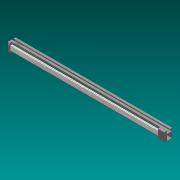
# Autodesk Inventor part: 连接桥
Saved by Autodesk Inventor 2021 (Build 250183000, 183)
## iProperties
Created: 2025-04-17
Part Number: 连接桥
Material: 常规
Document SubType Name: Modeling
Designer: 86155
Density: 1 g/cm^3
Appearance: 默认
Author: 86155
Autodesk Inventor part; units mm, degrees
ref_plane "YZ Plane" through (0, 0, 0) normal (1, 0, 0) x (0, 1, 0)
ref_plane "XZ Plane" through (0, 0, 0) normal (0, 1, 0) x (-1, 0, 0)
ref_plane "XY Plane" through (0, 0, 0) normal (0, 0, 1) x (1, 0, 0)
sketch "草图1" plane through (0, 0, 0) normal (1, 0, 0) x (0, 1, 0)
  line L0 (21, 12.5) -> (-21, 12.5)
  line L1 (-21, 12.5) -> (-21, -12.5)
  line L2 (-21, -12.5) -> (21, -12.5)
  line L3 (21, 12.5) -> (-21, -12.5) construction
  line L4 (-21, 12.5) -> (21, -12.5) construction
  line L5 (19, 10.5) -> (-19, 10.5)
  line L6 (-19, 10.5) -> (-19, -10.5)
  line L7 (-19, -10.5) -> (19, -10.5)
  line L8 (21, 4.5) -> (19, 4.5)
  line L9 (21, -4.5) -> (19, -4.5)
  line L10 (21, -12.5) -> (21, -4.5)
  line L11 (21, 4.5) -> (21, 12.5)
  line L12 (19, -10.5) -> (19, -4.5)
  line L13 (19, 4.5) -> (19, 10.5)
  line L14 (0, 10.5) -> (-2, 10.5)
  line L15 (-2, -10.5) -> (0, -10.5)
  line L16 (8, -12.5) -> (6, -12.5)
  line L17 (6, -12.5) -> (6, 12.5)
  line L18 (6, 12.5) -> (8, 12.5)
  line L19 (8, 12.5) -> (8, -12.5)
  point P0 (0, 0)
  point P1 (6, -10.5)
  point P2 (6, 10.5)
  point P3 (8, -10.5)
  point P4 (8, 10.5)
  dimension "d0" = 42
  dimension "d1" = 25
  dimension "d3" = 8
  dimension "d4" = 8
  dimension "d9" = 2
  dimension "d10" = 25
  constraints: 40 end point, 9 parallel, 7 perpendicular, 3 horizontal, 3 midpoint, 3 point on line, 2 other
  measures "d0" distance of L2.end L1.end
  measures "d1" distance of L1.end L0.end
  measures "d3" distance between parallel lines of L2 L9
  measures "d4" distance between parallel lines of L0 L8
  measures "d9" distance of L17.end L18.end
  measures "d10" distance between parallel lines of L6 L17
extrude "拉伸2" add sketch "草图1" along normal blind 680 contours L11 L8 L13 L5 L19 L0 | L19 L5 L17 L0 | L17 L5 L6 L7 L2 L1 L0 | L19 L7 L17 L5 | L19 L2 L17 L7 | L7 L12 L9 L10 L2 L19
sketch "草图2" plane through (0, -19, -10.5) normal (0, 0, 1) x (1, 0, 0)
  circle A0 centre (617.3314, 19) radius 3.3235 projected
  circle A1 centre (647.3314, 19) radius 3.3235 projected
  point P0 (0, 19)
extrude "拉伸3" cut sketch "草图2" against normal blind 2
sketch "草图3" plane through (0, 0, 0) normal (-1, 0, 0) x (0, 0, 1)
  line L0 (-12.5, 21) -> (-4.5, 21) projected
  line L1 (-12.5, -21) -> (-12.5, 21) projected
  line L2 (12.5, -21) -> (-12.5, -21) projected
  line L3 (12.5, 21) -> (12.5, -21) projected
  line L4 (4.5, 21) -> (12.5, 21) projected
  line L5 (4.5, 19) -> (4.5, 21) projected
  line L6 (10.5, 19) -> (4.5, 19) projected
  line L7 (10.5, 8) -> (10.5, 19) projected
  line L8 (-10.5, 8) -> (10.5, 8) projected
  line L9 (-10.5, 19) -> (-10.5, 8) projected
  line L10 (-4.5, 19) -> (-10.5, 19) projected
  line L11 (-4.5, 21) -> (-4.5, 19) projected
  line L12 (-10.5, 6) -> (-10.5, -19) projected
  line L13 (10.5, 6) -> (-10.5, 6) projected
  line L14 (10.5, -19) -> (10.5, 6) projected
  line L15 (-10.5, -19) -> (10.5, -19) projected
  line L16 (-10.5, 8) -> (-10.5, 6)
  line L17 (-10.5, 8) -> (10.5, 8) projected
  line L18 (10.5, -19) -> (10.5, 6) projected
  line L19 (10.5, 8) -> (10.5, 6)
  point P0 (0, 0)
  constraints: 4 end point, 1 collinear
extrude "拉伸4" add sketch "草图3" along normal blind 40 contours L0 L11 L10 L9 L16 L12 L15 L14 L19 L7 L6 L5 L4 L3 L2 L1
sketch "草图4" plane through (680, -21, 12.5) normal (0, 0, 1) x (1, 0, 0)
  circle A0 centre (-698, 21) radius 4.25
  line L0 (-720, 0) -> (-720, 42) projected
  point P0 (-680, 21)
  dimension "d17" = 8.5
  dimension "d18" = 22
  constraints: 1 centre point
  measures "d17" diameter of A0
  measures "d18" distance from line of L0 A0.centre
extrude "拉伸5" cut sketch "草图4" against normal blind 40
sketch "草图5" plane through (-40, 0, 0) normal (-1, 0, 0) x (0, 0, 1)
  line L0 (4.5, 21) -> (12.5, 21) projected
  line L1 (12.5, 21) -> (22.5, 21)
  line L2 (22.5, 21) -> (22.5, -21)
  line L3 (22.5, -21) -> (12.5, -21)
  line L4 (12.5, -21) -> (12.5, 21)
  point P0 (0, 0)
  dimension "d21" = 10
  dimension "d22" = 42
  constraints: 8 end point, 2 parallel, 1 horizontal, 1 perpendicular
  measures "d21" distance of L2.end L3.end
  measures "d22" distance of L1.end L2.end
extrude "拉伸6" add sketch "草图5" against normal blind 10
chamfer "倒角1" distance 2 angle 45 2 edges at (-35, 21, 22.5) (-35, -21, 22.5)
sketch "草图6" plane through (-30, 0, 0) normal (1, 0, 0) x (0, 0, -1)
  line L0 (-12.5, 21) -> (-12.5, -21) projected
  line L1 (-20.5, -10) -> (-20.5, 10)
  line L2 (-12.5, 10) -> (-12.5, -10)
  line L3 (-12.5, 21) -> (-20.5, 21) projected
  line L4 (-15.5, -10) -> (-15.5435, -10)
  line L5 (-15.5, -10) -> (-17.5, -10)
  line L6 (-17.5, -10) -> (-17.5, -7)
  line L7 (-17.5, -7) -> (-15.5, -7)
  line L8 (-15.5, -7) -> (-15.5, -10)
  line L9 (-15.5, 10) -> (-15.5, 7)
  line L10 (-15.5, 7) -> (-17.5, 7)
  line L11 (-17.5, 7) -> (-17.5, 10)
  line L12 (-20.5, 10) -> (-17.5, 10)
  line L13 (-15.5, 10) -> (-12.5, 10)
  line L14 (-12.5, -10) -> (-15.5, -10)
  line L15 (-17.5, -10) -> (-20.5, -10)
  point P0 (0, 0)
  dimension "d30" = 8
  dimension "d31" = 3
  dimension "d32" = 2
  dimension "d35" = 2
  constraints: 28 end point, 8 parallel, 4 horizontal, 3 perpendicular, 1 point on line
  measures "d30" distance between parallel lines of L0 L1
  measures "d31" distance between parallel lines of L1 L6
  measures "d32" distance between parallel lines of L8 L6
  measures "d35" distance between parallel lines of L11 L9
extrude "拉伸7" add sketch "草图6" along normal blind 680 contours L0 L14 L8 L7 L6 L15 L1 L12 L11 L10 L9 L13
sketch "草图7" plane through (650, 0, 0) normal (1, 0, 0) x (0, 0, -1)
  line L0 (-15.5, 10) -> (-12.5, 10) projected
  line L1 (-12.5, 21) -> (-12.5, 10) projected
  line L2 (-12.5, 21) -> (-20.5, 21) projected
  line L3 (-22.5, 19) -> (-20.5, 21) projected
  line L4 (-22.5, 19) -> (-22.5, -19) projected
  line L5 (-20.5, -21) -> (-22.5, -19) projected
  line L6 (-20.5, -21) -> (-12.5, -21) projected
  line L7 (-12.5, -10) -> (-12.5, -21) projected
  line L8 (-12.5, -10) -> (-15.5, -10) projected
  line L9 (-15.5, -10) -> (-15.5, -7) projected
  line L10 (-15.5, -7) -> (-17.5, -7) projected
  line L11 (-17.5, -7) -> (-17.5, -10) projected
  line L12 (-17.5, -10) -> (-20.5, -10) projected
  line L13 (-20.5, -10) -> (-20.5, 10) projected
  line L14 (-20.5, 10) -> (-17.5, 10) projected
  line L15 (-17.5, 10) -> (-17.5, 7) projected
  line L16 (-17.5, 7) -> (-15.5, 7) projected
  line L17 (-15.5, 7) -> (-15.5, 10) projected
  line L18 (-12.5, 10) -> (-12.5, -10) projected
  line L19 (-12.5, 10) -> (-15.5, 10) projected
  line L20 (-15.5, 10) -> (-15.5, 7) projected
  line L21 (-15.5, 7) -> (-17.5, 7) projected
  line L22 (-17.5, 7) -> (-17.5, 10) projected
  line L23 (-17.5, 10) -> (-20.5, 10) projected
  line L24 (-20.5, 10) -> (-20.5, -10) projected
  line L25 (-20.5, -10) -> (-17.5, -10) projected
  line L26 (-17.5, -10) -> (-17.5, -7) projected
  line L27 (-17.5, -7) -> (-15.5, -7) projected
  line L28 (-15.5, -7) -> (-15.5, -10) projected
  line L29 (-15.5, -10) -> (-12.5, -10) projected
  point P0 (0, 0)
extrude "拉伸8" add sketch "草图7" along normal blind 30
